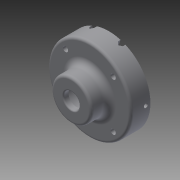
# Autodesk Inventor part: motorSupport-ExFlex-Part1
Saved by Autodesk Inventor 2014 SP2 (Build 180246200, 246)
## iProperties
Created: 2020-04-11
Part Number: motorSupport-ExFlex-Part1
Material: Generic
Document SubType Name: Sheet Metal
Designer: GauchoHP
Density: 1 g/cm^3
Sheet Metal Rule: Default_mm
Appearance: Default
Author: GauchoHP
Autodesk Inventor part; units mm, degrees
ref_plane "YZ Plane" through (0, 0, 0) normal (1, 0, 0) x (0, 1, 0)
ref_plane "XZ Plane" through (0, 0, 0) normal (0, 1, 0) x (-1, 0, 0)
ref_plane "XY Plane" through (0, 0, 0) normal (0, 0, 1) x (1, 0, 0)
sketch "Sketch1" plane through (0, 0, 0) normal (0, 1, 0) x (-1, 0, 0)
  circle A0 centre (0, 0) radius 6
  circle A1 centre (0, 0) radius 15.5
  dimension "d0" = 12
  dimension "d1" = 31
  constraints: 2 centre point, 2 coincident
  measures "d0" diameter of A0
  measures "d1" diameter of A1
extrude "Extrusion1" add sketch "Sketch1" along normal blind 4
sketch "Sketch2" plane through (0, 4, 0) normal (0, 1, 0) x (1, 0, 0)
  circle A0 centre (0, 0) radius 15.5 projected
  circle A1 centre (0, 0) radius 11.5
  dimension "d4" = 23
  constraints: 1 centre point, 1 coincident
  measures "d4" diameter of A1
extrude "Extrusion2" add sketch "Sketch2" along normal blind 10
sketch "Sketch3" plane through (0, 14, 0) normal (0, 1, 0) x (1, 0, 0)
  circle A0 centre (0, 0) radius 15.5 projected
  circle A1 centre (0, 0) radius 13
  circle A2 centre (0, 0) radius 32
  dimension "d8" = 26
  dimension "d9" = 64
  constraints: 2 centre point, 2 coincident
  measures "d8" diameter of A1
  measures "d9" diameter of A2
extrude "Extrusion3" add sketch "Sketch3" along normal blind 15 contours A0 | A2
sketch "Sketch4" plane through (0, 29, 0) normal (0, 1, 0) x (1, 0, 0)
  circle A0 centre (0, 0) radius 13 projected
  circle A1 centre (0, 0) radius 32 projected
  line L0 (-27, 3) -> (27, 3)
  line L1 (27, 3) -> (27, -3)
  line L2 (27, -3) -> (-27, -3)
  line L3 (-27, -3) -> (-27, 3)
  line L4 (-29, -3.5) -> (-16, -3.5)
  line L5 (-16, -3.5) -> (-16, 3.5)
  line L6 (-16, 3.5) -> (-29, 3.5)
  line L7 (-29, 3.5) -> (-29, -3.5)
  line L8 (16, 3.5) -> (29, 3.5)
  line L9 (29, 3.5) -> (29, -3.5)
  line L10 (29, -3.5) -> (16, -3.5)
  line L11 (16, -3.5) -> (16, 3.5)
  dimension "d12" = 6
  dimension "d13" = 3
  dimension "d14" = 54
  dimension "d15" = 27
  dimension "d16" = 13
  dimension "d17" = 7
  dimension "d18" = 3.5
  dimension "d19" = 16
  dimension "d20" = 13
  dimension "d21" = 7
  dimension "d22" = 3.5
  dimension "d23" = 16
  constraints: 24 end point, 6 parallel, 3 horizontal, 3 perpendicular
  measures "d12" distance of L0.end L1.end
  measures "d13" distance from line of A0.centre L0
  measures "d14" distance of L0.start L0.end
  measures "d15" distance from line of A0.centre L1
  measures "d16" distance of L6.end L5.end
  measures "d17" distance of L5.end L4.end
  measures "d18" distance from line of L6 A0.centre
  measures "d19" distance from line of L5 A0.centre
  measures "d20" distance of L9.end L10.end
  measures "d21" distance of L10.end L8.start
  measures "d22" distance from line of A0.centre L8
  measures "d23" distance from line of A0.centre L11
extrude "Extrusion4" cut sketch "Sketch4" against normal blind 9 contours A0 L2 L0 | A0 L0 L11 L2 | A0 L2 L5 L0 | L11 L8 L9 L10 L2 L1 L0 | L0 L1 L2 L11 | L5 L2 L3 L0 | L0 L3 L2 L5 L4 L7 L6
sketch "Sketch5" plane through (0, 20, 0) normal (0, 1, 0) x (1, 0, 0)
  line L0 (-16, 3) -> (-29, 3)
  line L1 (-29, 3) -> (-29, 3.5)
  line L2 (-29, 3.5) -> (-16, 3.5)
  line L3 (-16, 3.5) -> (-16, 3)
  line L4 (-16, -3) -> (-29, -3)
  line L5 (-29, -3) -> (-29, -3.5)
  line L6 (-29, -3.5) -> (-16, -3.5)
  line L7 (-16, -3.5) -> (-16, -3)
  constraints: 16 end point, 4 parallel, 2 horizontal, 2 perpendicular
extrude "Extrusion5" add sketch "Sketch5" along normal blind 2
sketch "Sketch6" plane through (0, 20, 0) normal (0, 1, 0) x (1, 0, 0)
  line L0 (16, 3) -> (29, 3)
  line L1 (29, 3) -> (29, 3.5)
  line L2 (29, 3.5) -> (16, 3.5)
  line L3 (16, 3.5) -> (16, 3)
  line L4 (16, -3) -> (29, -3)
  line L5 (29, -3) -> (29, -3.5)
  line L6 (29, -3.5) -> (16, -3.5)
  line L7 (16, -3.5) -> (16, -3)
  constraints: 16 end point, 4 parallel, 2 horizontal, 2 perpendicular
extrude "Extrusion6" add sketch "Sketch6" along normal blind 2
sketch "Sketch7" plane through (29, 29, -3.5) normal (-1, 0, 0) x (0, 0, 1)
  line L0 (0, 0) -> (7, 0) projected
  line L1 (0, 0) -> (0, -7) projected
  circle A0 centre (3.5, -3.5) radius 1.5
  point P0 (3.5, -29)
  dimension "d30" = 3
  dimension "d31" = 7
  dimension "d32" = 3.5
  dimension "d33" = 3.5
  constraints: 1 centre point
  measures "d30" diameter of A0
  measures "d31" distance of L0.start L1.end
  measures "d32" distance from line of L0 A0.centre
  measures "d33" distance from line of A0.centre L1
extrude "Extrusion7" cut sketch "Sketch7" against normal blind 3
sketch "Sketch8" plane through (-29, 29, 3.5) normal (1, 0, 0) x (0, 0, -1)
  line L0 (0, 0) -> (7, 0) projected
  line L1 (0, 0) -> (0, -7) projected
  circle A0 centre (3.5, -3.5) radius 1.5
  point P0 (3.5, -29)
  dimension "d36" = 3
  dimension "d37" = 3.5
  dimension "d39" = 3.5
  constraints: 1 centre point
  measures "d36" diameter of A0
  measures "d37" distance from line of L0 A0.centre
  measures "d39" distance from line of A0.centre L1
extrude "Extrusion8" cut sketch "Sketch8" against normal blind 3
sketch "Sketch9" plane through (0, 14, 0) normal (0, -1, 0) x (1, 0, 0)
  circle A0 centre (0, 0) radius 15.5 projected
  circle A1 centre (0, 0) radius 26
  line L0 (-18.3848, -18.3848) -> (18.3848, 18.3848)
  line L1 (-18.3848, 18.3848) -> (18.3848, -18.3848)
  circle A2 centre (-18.3848, 18.3848) radius 2
  circle A3 centre (18.3848, 18.3848) radius 2
  circle A4 centre (18.3848, -18.3848) radius 2
  circle A5 centre (-18.3848, -18.3848) radius 2
  dimension "d42" = 52
  dimension "d43" = 4
  dimension "d44" = 4
  dimension "d45" = 4
  dimension "d46" = 4
  constraints: 5 centre point, 5 coincident, 4 end point
  measures "d42" diameter of A1
  measures "d43" diameter of A2
  measures "d44" diameter of A3
  measures "d45" diameter of A4
  measures "d46" diameter of A5
extrude "Extrusion9" cut sketch "Sketch9" against normal blind 25 contours A3 A1 L0 | L0 A1 A3 | A4 A1 L1 | L1 A1 A4 | A2 A1 L1 | L1 A1 A2 | A1 A3 | A5 A1 L0 | L0 A1 A5 | A1 A4 | A1 A2 | A1 A5
fillet "Fillet1" radius 2 1 edges at (-32, 14, 0)
fillet "Fillet2" radius 5 1 edges at (-15.5, 14, 0)
fillet "Fillet3" radius 2 1 edges at (15.5, 0, 0)
fillet "Fillet4" radius 1 1 edges at (6, 0, 0)
sketch "Sketch10" plane through (0, 29, 0) normal (0, 1, 0) x (1, 0, 0)
  circle A0 centre (0, 0) radius 32 projected
  arc A1 (-12.6491, -3) -> (12.6491, -3) centre (0, 0) ccw projected
  arc A2 (12.6491, 3) -> (-12.6491, 3) centre (0, 0) ccw projected
  line L0 (-6.2727, 11.3865) -> (-12.8026, 29.3273)
  line L1 (-4.4463, 12.216) -> (-10.9446, 30.0702)
  line L2 (-2.5139, 12.7546) -> (-9.0439, 30.6954)
  line L3 (2.4494, 12.7672) -> (8.9814, 30.7137)
  line L4 (6.2151, 11.4181) -> (12.743, 29.3533)
  line L5 (18.9742, -52.1313) -> (10.9446, -30.0702)
  line L6 (1.0296, -2.8289) -> (-1.0987, 3.0188)
  line L7 (9.0439, -30.6954) -> (2.5139, -12.7546)
  line L8 (-0.0346, -5.7527) -> (-2.1629, 0.0949)
  line L9 (12.8026, -29.3273) -> (6.2727, -11.3865)
  line L10 (2.0938, 0.0949) -> (-0.0346, 5.9426)
  line L11 (-9.1063, -30.677) -> (-2.5784, -12.7417)
  line L12 (-0.0346, -5.7527) -> (2.0938, 0.0949)
  line L13 (-1.0987, -2.8289) -> (1.0296, 3.0188)
  line L14 (-12.8622, -29.3012) -> (-6.3302, -11.3547)
  line L15 (-2.1629, 0.0949) -> (-0.0346, 5.9426)
  line L16 (-16, 3) -> (-12.6491, 3) projected
  arc A3 (-2.5139, 12.7546) -> (-6.2727, 11.3865) centre (0, 0) ccw
  arc A4 (-12.6491, 3) -> (2.4494, 12.7672) centre (0, 0) ccw
  arc A5 (-12.8622, -29.3012) -> (8.9814, 30.7137) centre (0, 0) ccw
  arc A6 (-9.0439, 30.6954) -> (-12.8026, 29.3273) centre (0, 0) ccw
  point P0 (-12.8026, 29.3273)
  dimension "d54" = 82.2014
  dimension "d55" = 29.9189
  constraints: 33 end point, 24 parallel, 20 point on circle, 4 centre point, 4 midpoint, 2 coincident, 1 point on line, 10 other
  measures "d54" vertical distance of L5.start L1.end
  measures "d55" horizontal distance of L5.start L1.end
extrude "Extrusion10" cut sketch "Sketch10" against normal blind 4 contours L4 A2 L3 A0 | A0 L7 A1 L9 | L2 A2 L1 A0 | L1 A2 L0 A0 | A0 L14 A1 L11
chamfer "Chamfer1" distance 2 angle 45 8 edges at (-9.5962, 25, 20.3279) (-5.8423, 25, 21.7094) (9.5377, 25, 20.3569) (5.7789, 25, 21.725) (9.479, 25, -20.3857) (5.7154, 25, -21.7405) (-5.7789, 25, -21.725) (-9.5377, 25, -20.3569)
equation "\"BendRadius\" = Thickness"
equation "\"BendReliefWidth\" = Thickness"
equation "\"BendReliefDepth\" = 0.5 * Thickness"
equation "\"CornerReliefSize\" = 4 * Thickness"
equation "\"MinimumRemnant\" = 2 * Thickness"
equation "\"TransitionRadius\" = BendRadius"
equation "\"JacobiRadiusSize\" = BendRadius"
equation "\"GapSize\" = Thickness"
equation "\"Thickness\" = 0.5"
body "Solid1"
